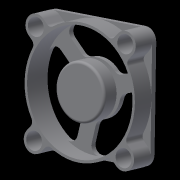
# Autodesk Inventor part: Fan12VDC
Saved by Autodesk Inventor 2015 (Build 190159000, 159)
## iProperties
Created: 2015-01-27
Part Number: Fan12VDC
Material: Generic
Document SubType Name: Modeling
Designer: Inventor
Mass: 6.16683 g
Surface Area: 72.8558 cm^2
Volume: 6.16683 cm^3
Density: 1 g/cm^3
Appearance: Default
RuleStatus: InUse
BeforeDocSave0: UpdateBoundingBox
Author: Inventor
Autodesk Inventor part; units mm, degrees
ref_plane "YZ Plane" through (0, 0, 0) normal (1, 0, 0) x (0, 1, 0)
ref_plane "XZ Plane" through (0, 0, 0) normal (0, 1, 0) x (-1, 0, 0)
ref_plane "XY Plane" through (0, 0, 0) normal (0, 0, 1) x (1, 0, 0)
sketch "Base" plane through (0, 0, 0) normal (0, 1, 0) x (-1, 0, 0)
  circle A0 centre (0, 0) radius 22.5 construction
  line L0 (22.5, 22.5) -> (-22.5, 22.5)
  line L1 (-22.5, 22.5) -> (-22.5, -22.5)
  line L2 (-22.5, -22.5) -> (22.5, -22.5)
  line L3 (22.5, -22.5) -> (22.5, 22.5)
  dimension "d0" = 45
  constraints: 8 end point, 4 tangent, 2 parallel, 1 centre point, 1 coincident, 1 horizontal, 1 perpendicular
  measures "d0" diameter of A0
extrude "BaseFeature" add sketch "Base" along normal blind 2
fillet "CornerFilletsFeature" radius 4.5 4 edges at (22.5, 1, -22.5) (-22.5, 1, -22.5) (22.5, 1, 22.5) (-22.5, 1, 22.5)
sketch "MountHoles" plane through (0, 2, 0) normal (0, 1, 0) x (1, 0, 0)
  line L0 (-18.25, 18.25) -> (18.25, 18.25) construction
  line L1 (18.25, 18.25) -> (18.25, -18.25) construction
  line L2 (18.25, -18.25) -> (-18.25, -18.25) construction
  line L3 (-18.25, -18.25) -> (-18.25, 18.25) construction
  line L4 (22.5, -18) -> (22.5, 18) projected
  line L5 (18, 22.5) -> (-18, 22.5) projected
  line L6 (-22.5, 18) -> (-22.5, -18) projected
  line L7 (-18, -22.5) -> (18, -22.5) projected
  dimension "d4" = 4.25
  dimension "d5" = 4.25
  dimension "d6" = 4.25
  dimension "d7" = 4.25
  constraints: 8 end point, 3 parallel, 1 horizontal, 1 perpendicular
  measures "d4" distance between parallel lines of L4 L1
  measures "d5" distance between parallel lines of L5 L0
  measures "d6" distance between parallel lines of L6 L3
  measures "d7" distance between parallel lines of L7 L2
hole "MountHolesFeature" at (18.25, 2, -18.25) at (-18.25, 2, -18.25) at (-18.25, 2, 18.25) at (18.25, 2, 18.25) direction (0, -1, 0) diameter 3 end through all
sketch "Shaft" plane through (0, 2, 0) normal (0, 1, 0) x (1, 0, 0)
  circle A0 centre (0, 0) radius 22.5 projected
  circle A1 centre (0, 0) radius 21.5
  dimension "d15" = 1
  constraints: 1 centre point, 1 coincident
  measures "d15" radial gap between concentric circles of A0 A1
extrude "ShaftFeature" cut sketch "Shaft" against normal through all contours A1
sketch "Top" plane through (0, 2, 0) normal (0, 1, 0) x (1, 0, 0)
  circle A0 centre (0, 0) radius 21.5
  circle A1 centre (0, 0) radius 22.5
  line L0 (18, 22.5) -> (-18, 22.5)
  circle A2 centre (18.25, 18.25) radius 3.257347
  circle A3 centre (-18.25, 18.25) radius 3.257347
  circle A4 centre (-18.25, -18.25) radius 3.257347
  circle A5 centre (18.25, -18.25) radius 3.257347
  circle A6 centre (18.25, 18.25) radius 4.257347
  circle A7 centre (-18.25, 18.25) radius 4.257347
  circle A8 centre (-18.25, -18.25) radius 4.257347
  circle A9 centre (18.25, -18.25) radius 4.257347
  line L1 (-15.239601, 21.260399) -> (-12.612101, 18.632898)
  line L2 (-21.260399, 15.239601) -> (-18.632898, 12.612101)
  line L3 (-18.25, 18.25) -> (0, 0) construction
  line L4 (0, 0) -> (18.25, 18.25) construction
  line L5 (15.239601, 21.260399) -> (12.612101, 18.632898)
  line L6 (21.260399, 15.239601) -> (18.632898, 12.612101)
  line L7 (-21.260399, -15.239601) -> (-18.632898, -12.612101)
  line L8 (-15.239601, -21.260399) -> (-12.612101, -18.632898)
  line L9 (0, 0) -> (-18.25, -18.25) construction
  line L10 (0, 0) -> (18.25, -18.25) construction
  line L11 (21.260399, -15.239601) -> (18.632898, -12.612101)
  line L12 (15.239601, -21.260399) -> (12.612101, -18.632898)
  circle A10 centre (18.25, -18.25) radius 1.5
  circle A11 centre (18.25, 18.25) radius 1.5
  circle A12 centre (-18.25, 18.25) radius 1.5
  circle A13 centre (-18.25, -18.25) radius 1.5
  point P0 (-18, -22.5)
  point P1 (18, -22.5)
  dimension "d21" = 1
  dimension "d22" = 1
  dimension "d23" = 1
  dimension "d24" = 1
  constraints: 24 end point, 12 point on circle, 8 centre point, 8 parallel, 8 tangent, 5 coincident, 4 concentric, 1 horizontal, 10 other
  measures "d21" radial gap between concentric circles of A9 A5
  measures "d22" radial gap between concentric circles of A6 A2
  measures "d23" radial gap between concentric circles of A7 A3
  measures "d24" radial gap between concentric circles of A8 A4
extrude "TopFeature" add sketch "Top" along normal blind 8 contours A1 A9 A8 A7 A6 | A1 A6 L6 | L11 A9 A1 | A6 A1 | A1 A6 | A9 A1 | A1 A9 | A1 L5 A6 | A9 L12 A1 | L8 A8 A1 | A1 A7 L1 | A7 A1 | A8 A1 | A1 A8 | A7 A1 | A7 A1 L2 | A8 L7 A1
fillet "TopFilletsFeature" radius 2 8 edges at (-12.6121, 6, -18.6329) (-18.6329, 6, -12.6121) (12.6121, 6, -18.6329) (18.6329, 6, -12.6121) (18.6329, 6, 12.6121) (12.6121, 6, 18.6329) (-12.6121, 6, 18.6329) (-18.6329, 6, 12.6121)
sketch "HeadMount" plane through (0, 0, 0) normal (0, -1, 0) x (1, 0, 0)
  circle A0 centre (0, 0) radius 21.5 construction
  line L0 (0, 0) -> (-5.38317, 20.815174) construction
  line L1 (0, 0) -> (20.718055, -5.745625) construction
  line L2 (0, 0) -> (-15.334885, -15.069549) construction
  circle A1 centre (0, 0) radius 10
  line L3 (0.51597, 9.98668) -> (-2.478727, 21.566314)
  line L4 (0.51597, 9.98668) -> (-5.292916, 8.4844)
  line L5 (-5.292916, 8.4844) -> (-8.287613, 20.064034)
  line L6 (-8.287613, 20.064034) -> (-2.478727, 21.566314)
  circle A2 centre (0, 0) radius 21.5
  line L7 (-31.5, 0) -> (31.5, 0) construction
  line L8 (8.390734, -5.440183) -> (9.994164, 0.3416)
  line L9 (9.994164, 0.3416) -> (21.51977, -2.854734)
  line L10 (21.51977, -2.854734) -> (19.91634, -8.636516)
  line L11 (19.91634, -8.636516) -> (8.390734, -5.440183)
  line L12 (-4.701248, -8.826) -> (-8.906703, -4.546497)
  line L13 (-8.906703, -4.546497) -> (-17.437612, -12.929798)
  line L14 (-17.437612, -12.929798) -> (-13.232157, -17.209301)
  line L15 (-13.232157, -17.209301) -> (-4.701248, -8.826)
  point P0 (-2.388473, 9.23554)
  point P1 (9.192449, -2.549292)
  point P2 (-6.803976, -6.686248)
  dimension "d26" = 120
  dimension "d27" = 120
  dimension "d28" = 20
  dimension "d30" = 6
  dimension "d31" = 15.5
  dimension "d32" = 6
  dimension "d33" = 6
  constraints: 30 end point, 8 perpendicular, 6 point on circle, 4 parallel, 3 midpoint, 3 point on line, 3 tangent, 1 centre point, 1 coincident
  measures "d26" angle of L1 L0
  measures "d27" angle of L2 L0
  measures "d28" diameter of A1
  measures "d30" distance of L5.end L3.end
  measures "d31" angle of L7 L1
  measures "d32" distance of L9.end L10.end
  measures "d33" distance of L13.end L14.end
extrude "HeadMountFeature" add sketch "HeadMount" against normal blind 2 contours A1 L8 | A1 L9 A2 L11 | L8 A1 L12 L4 | L4 A1 | A2 L5 L6 | A1 L5 A2 L3 | L9 L10 A2 | L15 A2 L13 A1 | A1 L12 | A2 L10 L11 | A2 L6 L3 | L15 L14 A2 | A2 L14 L13
fillet "HeadMountFilletsFeature" radius 3 12 edges at (19.7137, 1, -8.5803) (21.3171, 1, -2.7985) (-17.2876, 1, -12.7824) (-13.0821, 1, -17.0619) (-2.4261, 1, 21.3627) (-8.235, 1, 19.8604) (-8.9067, 1, -4.5465) (-4.7012, 1, -8.826) (8.3907, 1, -5.4402) (9.9942, 1, 0.3416) (0.516, 1, 9.9867) (-5.2929, 1, 8.4844)
sketch "HeadStem" plane through (0, 2, 0) normal (0, 1, 0) x (1, 0, 0)
  arc A0 (-9.562355, 2.925983) -> (-6.689545, -7.433033) centre (0, 0) ccw
  circle A1 centre (0, 0) radius 6
  dimension "d37" = 12
  constraints: 1 centre point, 1 coincident
  measures "d37" diameter of A1
extrude "HeadStemFeature" add sketch "HeadStem" along normal blind 2
sketch "Head" plane through (0, 4, 0) normal (0, 1, 0) x (1, 0, 0)
  circle A0 centre (0, 0) radius 6 projected
  circle A1 centre (0, 0) radius 10
  dimension "d40" = 20
  constraints: 1 centre point, 1 coincident
  measures "d40" diameter of A1
extrude "HeadFeature" add sketch "Head" along normal up to surface (6 mm away) separate body contours A0 | A1
fillet "HeadTopFilletFeature" radius 1 1 edges at (-10, 10, 0)
equation "\"d5\" = d4"
equation "\"d6\" = d4"
equation "\"d7\" = d4"
body "Solid1"
body "Solid2"
